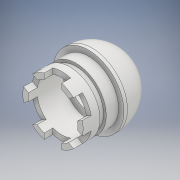
# Autodesk Inventor part: STK00-002
Saved by Autodesk Inventor 2018 (Build 220112000, 112)
## iProperties
Created: 2018-02-13
Part Number: STK00-002
Material: ABS Plastic
Document SubType Name: Modeling
Designer: JARVIS
Density: 1.06 g/cm^3
Appearance: Smooth - White
Mass: 17.72 g
Surface Area: 76.9077 cm^2
Volume: 16.717 cm^3
Author: JARVIS
Autodesk Inventor part; units mm, degrees
ref_plane "YZ Plane" through (0, 0, 0) normal (1, 0, 0) x (0, 1, 0)
ref_plane "XZ Plane" through (0, 0, 0) normal (0, 1, 0) x (-1, 0, 0)
ref_plane "XY Plane" through (0, 0, 0) normal (0, 0, 1) x (1, 0, 0)
sketch "Sketch1" plane through (0, 0, 0) normal (0, 0, 1) x (1, 0, 0)
  line L0 (20, 2) -> (20, 0)
  line L1 (20, 0) -> (17, 0)
  line L2 (17, 0) -> (17, -20)
  line L3 (17, -20) -> (14, -20)
  line L4 (14, -20) -> (14, 0)
  line L5 (14, 0) -> (0, 0)
  arc A0 (20, 2) -> (0, 21.7641) centre (0, 1.7627) ccw
  line L6 (0, 0) -> (0, 21.7641)
  point P0 (0, 0)
  point P1 (0, 0)
  dimension "d0" = 3
  dimension "d1" = 2
  dimension "d3" = 20
  dimension "d22" = 3
  dimension "d23" = 20
  constraints: 14 end point, 4 coincident, 4 perpendicular, 2 point on circle, 2 vertical alignment, 1 centre point, 1 point on line
  measures "d0" distance of L2.end L3.end
  measures "d1" distance of L0.start L0.end
  measures "d3" distance of L1.end L2.end
  measures "d22" distance of L0.end L1.end
  measures "d23" distance of point (0, 0) L0.end
revolve "Revolution1" add sketch "Sketch1" angle 360 about axis through (0, 0, 0) along (0, 1, 0)
sketch "Sketch2" plane through (0, 0, 0) normal (0, 0, 1) x (1, 0, 0)
  line L0 (-5, -35) -> (5, -35)
  line L1 (5, -35) -> (5, -15)
  line L2 (5, -15) -> (-5, -15)
  line L3 (-5, -15) -> (-5, -35)
  line L4 (-20, 0) -> (20, 0) projected
  point P0 (0, 0)
  point P1 (0, -35)
  point P2 (0, 0)
  dimension "d7" = 10
  dimension "d8" = 15
  dimension "d9" = 20
  constraints: 8 end point, 2 midpoint, 2 parallel, 1 horizontal, 1 perpendicular, 1 vertical alignment
  measures "d7" distance of L0.start L0.end
  measures "d8" distance between parallel lines of L2 L4
  measures "d9" distance of L0.end L1.end
extrude "Extrusion1" cut sketch "Sketch2" along normal through all both and the other way through all
pattern_circular "Circular Pattern1" count 6 over 360 about axis through (0, -10, 0) along (0, 1, 0) of "Extrusion1"
sketch "Sketch3" plane through (0, 0, 0) normal (0, -1, 0) x (1, 0, 0)
  circle A0 centre (0, 0) radius 10
  point P0 (0, 0)
  dimension "d15" = 20
  constraints: 1 centre point, 1 coincident
  measures "d15" diameter of A0
extrude "Extrusion2" cut sketch "Sketch3" against normal blind 15.5
sketch "Sketch4" plane through (0, 0, 0) normal (0, 0, 1) x (1, 0, 0)
  line L0 (19.1095, -7) -> (15.5, -7)
  line L1 (15.5, -7) -> (15.5, -10.5)
  line L2 (15.5, -10.5) -> (19.1095, -10.5)
  line L3 (19.1095, -10.5) -> (19.1095, -7)
  line L4 (17, 0) -> (17, -20) projected
  line L5 (0, -24) -> (0, 4) projected
  line L6 (-20, 0) -> (20, 0) projected
  point P0 (0, 0)
  dimension "d18" = 1.5
  dimension "d19" = 3.5
  dimension "d21" = 7
  constraints: 8 end point, 2 parallel, 1 horizontal, 1 perpendicular
  measures "d18" distance between parallel lines of L1 L4
  measures "d19" distance of L2.end L0.start
  measures "d21" distance between parallel lines of L0 L6
revolve "Revolution2" cut sketch "Sketch4" angle 360 about axis through (0, -10, 0) along (0, 1, 0)
body "Solid1"
